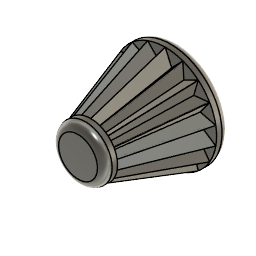
air filter (Autodesk Fusion 360 design; units mm, degrees)
part number: 2026-06-07-15-33-17-736
Autodesk Fusion 360 part; units mm, degrees
sketch "Sketch1" plane through (0, 0, 0) normal (0, 1, 0) x (1, 0, 0)
  line L0 (0, 0) -> (0, -70) construction
  line L1 (0, 0) -> (-8.8163, -50)
  line L2 (-8.8163, -50) -> (0, -70)
  line L3 (8.8163, -50) -> (0, -70)
  line L4 (0, 0) -> (8.8163, -50)
  dimension "d1" = 70
  dimension "d2" = 10
  dimension "d3" = 50
  dimension "d4" = 20
  constraint coincident L0.start L1.start
  constraint vertical L0
  constraint symmetric L1.start L0 L4.start
  constraint symmetric L2.end L0 L3.end
  constraint symmetric L0 L1.end L3.start
  measures "d1" distance of L0.start L0.end
  measures "d2" angle of L0 L1
  measures "d3" vertical distance of L0.start L1.end
  measures "d4" vertical distance of L0.end L1.end
ref_plane "WorkPlane1" through (0, -101.5, 0) normal (0, 1, 0) x (0, 0, 1)
sketch "Sketch2" plane through (0, -101.5, 0) normal (0, 1, 0) x (1, 0, 0)
  line L0 (0, 0) -> (0, -36.5) construction
  line L1 (0, 0) -> (-4.4082, -25)
  line L2 (-4.4082, -25) -> (0, -36.5)
  line L3 (4.4082, -25) -> (0, -36.5)
  line L4 (0, 0) -> (4.4082, -25)
  dimension "d6" = 36.5
  dimension "d7" = 10
  dimension "d8" = 25
  dimension "d9" = 11.5
  constraint coincident L0.start L1.start
  constraint vertical L0
  constraint symmetric L1.start L0 L4.start
  constraint symmetric L2.end L0 L3.end
  constraint symmetric L0 L1.end L3.start
  measures "d6" distance of L0.start L0.end
  measures "d7" angle of L0 L1
  measures "d8" vertical distance of L0.start L1.end
  measures "d9" vertical distance of L0.end L1.end
loft "Loft1" add profiles "Sketch1", "Sketch2" section 1 section 2 makes body 1
pattern_circular "C-Pattern1" count 18 over 360 about axis through (0, 0, 0) along (0, -1, 0) of bodies 1 makes body 2 at (-4.0408, -16.9167, 22.9167) makes body 3 at (-26.7089, -33.8333, 39.4504) makes body 4 at (-38.591, -33.8333, 27.9362) makes body 5 at (-45.8184, -33.8333, 13.0526) makes body 6 at (-53.5858, -16.9167, -13.5518) makes body 7 at (-43.489, -33.8333, -19.4527) makes body 8 at (-32.3382, -16.9167, -44.8256) makes body 9 at (-15.0567, -16.9167, -53.1826) makes body 10 at (4.0408, -16.9167, -55.125) makes body 11 at (11.6054, -33.8333, -46.2062) makes body 12 at (26.7089, -33.8333, -39.4504) makes body 13 at (49.7601, -16.9167, -24.063) makes body 14 at (54.9892, -16.9167, -5.5929) makes body 15 at (47.5195, -33.8333, 3.4054) makes body 16 at (45.7192, -16.9167, 31.062) makes body 17 at (32.3382, -16.9167, 44.8256) makes body 18 at (4.0408, -16.9167, 22.9167)
combine "Combine1" operation add target body 1 tool bodies 2 3 4 5 6 7 8 9 10 11 12 13 14 15 16 17 18
shell "Shell1" thickness 1 removed faces 2 at (-1.2922, -101.5, -7.3282) at (0, 0, 0) on bodies 1
sketch "Sketch3" plane through (0, 0, 0) normal (0, 1, 0) x (1, 0, 0)
  circle A0 centre (0, 0) radius 70
  dimension "d13" = 140
  constraint coincident A0.centre origin
  measures "d13" diameter of A0
extrude "Extrude1" add sketch "Sketch3" along normal blind 17.35 bodies 1
sketch "Sketch4" plane through (0, -101.5, 0) normal (0, -1, 0) x (1, 0, 0)
  line L0 (-11.5213, 31.6544) -> (-4.0679, 23.0702)
  line L1 (-4.0679, 23.0702) -> (0, 33.686)
  line L2 (0, 33.686) -> (4.0679, 23.0702)
  line L3 (4.0679, 23.0702) -> (11.5213, 31.6544)
  line L4 (11.5213, 31.6544) -> (11.7131, 20.2876)
  line L5 (11.7131, 20.2876) -> (21.6529, 25.8049)
  line L6 (21.6529, 25.8049) -> (17.9455, 15.058)
  line L7 (17.9455, 15.058) -> (29.1729, 16.843)
  line L8 (29.1729, 16.843) -> (22.0134, 8.0122)
  line L9 (22.0134, 8.0122) -> (33.1742, 5.8495)
  line L10 (33.1742, 5.8495) -> (23.4261, 0)
  line L11 (23.4261, 0) -> (33.1742, -5.8495)
  line L12 (33.1742, -5.8495) -> (22.0134, -8.0122)
  line L13 (22.0134, -8.0122) -> (29.1729, -16.843)
  line L14 (29.1729, -16.843) -> (17.9455, -15.058)
  line L15 (17.9455, -15.058) -> (21.6529, -25.8049)
  line L16 (21.6529, -25.8049) -> (11.7131, -20.2876)
  line L17 (11.7131, -20.2876) -> (11.5213, -31.6544)
  line L18 (11.5213, -31.6544) -> (4.0679, -23.0702)
  line L19 (4.0679, -23.0702) -> (0, -33.686)
  line L20 (0, -33.686) -> (-4.0679, -23.0702)
  line L21 (-4.0679, -23.0702) -> (-11.5213, -31.6544)
  line L22 (-11.5213, -31.6544) -> (-11.7131, -20.2876)
  line L23 (-11.7131, -20.2876) -> (-21.6529, -25.8049)
  line L24 (-21.6529, -25.8049) -> (-17.9455, -15.058)
  line L25 (-17.9455, -15.058) -> (-29.1729, -16.843)
  line L26 (-29.1729, -16.843) -> (-22.0134, -8.0122)
  line L27 (-22.0134, -8.0122) -> (-33.1742, -5.8495)
  line L28 (-33.1742, -5.8495) -> (-23.4261, 0)
  line L29 (-23.4261, 0) -> (-33.1742, 5.8495)
  line L30 (-33.1742, 5.8495) -> (-22.0134, 8.0122)
  line L31 (-22.0134, 8.0122) -> (-29.1729, 16.843)
  line L32 (-29.1729, 16.843) -> (-17.9455, 15.058)
  line L33 (-17.9455, 15.058) -> (-21.6529, 25.8049)
  line L34 (-21.6529, 25.8049) -> (-11.7131, 20.2876)
  line L35 (-11.7131, 20.2876) -> (-11.5213, 31.6544)
  line L36 (4.4082, 25) -> (0, 36.5)
  line L37 (0, 36.5) -> (-4.4082, 25)
  line L38 (-4.4082, 25) -> (-12.4837, 34.2988)
  line L39 (-12.4837, 34.2988) -> (-12.6928, 21.9846)
  line L40 (-12.6928, 21.9846) -> (-23.4617, 27.9606)
  line L41 (-23.4617, 27.9606) -> (-19.4465, 16.3176)
  line L42 (-19.4465, 16.3176) -> (-31.6099, 18.25)
  line L43 (-31.6099, 18.25) -> (-23.8547, 8.6824)
  line L44 (-23.8547, 8.6824) -> (-35.9455, 6.3382)
  line L45 (-35.9455, 6.3382) -> (-25.3857, 0)
  line L46 (-25.3857, 0) -> (-35.9455, -6.3382)
  line L47 (-35.9455, -6.3382) -> (-23.8547, -8.6824)
  line L48 (-23.8547, -8.6824) -> (-31.6099, -18.25)
  line L49 (-31.6099, -18.25) -> (-19.4465, -16.3176)
  line L50 (-19.4465, -16.3176) -> (-23.4617, -27.9606)
  line L51 (-23.4617, -27.9606) -> (-12.6928, -21.9846)
  line L52 (-12.6928, -21.9846) -> (-12.4837, -34.2988)
  line L53 (-12.4837, -34.2988) -> (-4.4082, -25)
  line L54 (-4.4082, -25) -> (0, -36.5)
  line L55 (0, -36.5) -> (4.4082, -25)
  line L56 (4.4082, -25) -> (12.4837, -34.2988)
  line L57 (12.4837, -34.2988) -> (12.6928, -21.9846)
  line L58 (12.6928, -21.9846) -> (23.4617, -27.9606)
  line L59 (23.4617, -27.9606) -> (19.4465, -16.3176)
  line L60 (19.4465, -16.3176) -> (31.6099, -18.25)
  line L61 (31.6099, -18.25) -> (23.8547, -8.6824)
  line L62 (23.8547, -8.6824) -> (35.9455, -6.3382)
  line L63 (35.9455, -6.3382) -> (25.3857, 0)
  line L64 (25.3857, 0) -> (35.9455, 6.3382)
  line L65 (35.9455, 6.3382) -> (23.8547, 8.6824)
  line L66 (23.8547, 8.6824) -> (31.6099, 18.25)
  line L67 (31.6099, 18.25) -> (19.4465, 16.3176)
  line L68 (19.4465, 16.3176) -> (23.4617, 27.9606)
  line L69 (23.4617, 27.9606) -> (12.6928, 21.9846)
  line L70 (12.6928, 21.9846) -> (12.4837, 34.2988)
  line L71 (12.4837, 34.2988) -> (4.4082, 25)
  circle A0 centre (0, 0) radius 36.5
  dimension "d16" = 73
  constraint coincident A0.centre origin
  measures "d16" diameter of A0
extrude "Extrude2" add sketch "Sketch4" along normal blind 17.35 contours L0 L1 L2 L3 L4 L5 L6 L7 L8 L9 L10 L11 L12 L13 L14 L15 L16 L17 L18 L19 L20 L21 L22 L23 L24 L25 L26 L27 L28 L29 L30 L31 L32 L33 L34 L35 | L36 L37 L38 L39 L40 L41 L42 L43 L44 L45 L46 L47 L48 L49 L50 L51 L52 L53 L54 L55 L56 L57 L58 L59 L60 L61 L62 L63 L64 L65 L66 L67 L68 L69 L70 L71 | L36 L71 A0 | L37 L38 A0 | L69 L70 A0 | L39 L40 A0 | L67 L68 A0 | L41 L42 A0 | L65 L66 A0 | L43 L44 A0 | L63 L64 A0 | L45 L46 A0 | L47 L48 A0 | L61 L62 A0 | L49 L50 A0 | L59 L60 A0 | L51 L52 A0 | L57 L58 A0 | L53 L54 A0 | L55 L56 A0 bodies 1
fillet "Fillet1" radius 10 2 edges at (-34.0299, -118.85, -13.199) (-65.2629, 17.35, 25.3131) on bodies 1
sketch "Sketch5" plane through (0, 17.35, 0) normal (0, 1, 0) x (-1, 0, 0)
  circle A0 centre (0, 0) radius 60
  circle A1 centre (0, 0) radius 10
  dimension "d21" = 20
  constraint coincident A0.centre A1.centre
  measures "d21" diameter of A1
extrude "Extrude3" cut sketch "Sketch5" against normal blind 30 contours A1 bodies 1
